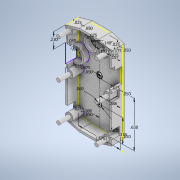
# Autodesk Inventor part: Back half gearbox
Saved by Autodesk Inventor 2020 (Build 240168000, 168)
## iProperties
Created: 2022-05-09
Part Number: Back half gearbox
Material: Generic
Document SubType Name: Modeling
Designer: Administrator
Density: 1 g/cm^3
Appearance: Default
Author: Administrator
Autodesk Inventor part; units mm, degrees
ref_plane "YZ Plane" through (0, 0, 0) normal (1, 0, 0) x (0, 1, 0)
ref_plane "XZ Plane" through (0, 0, 0) normal (0, 1, 0) x (-1, 0, 0)
ref_plane "XY Plane" through (0, 0, 0) normal (0, 0, 1) x (1, 0, 0)
sketch "Sketch1" plane through (0, 0, 0) normal (0, 0, 1) x (1, 0, 0)
  line L0 (-4.445, 2.3537) -> (-11.2171, 2.3537)
  line L1 (-16.0528, 3.6237) -> (-16.0528, 32.5162)
  line L2 (-11.2171, 33.8978) -> (-4.445, 33.8978)
  line L3 (0, 32.5162) -> (0, 3.6237)
  line L4 (-16.0528, 32.5162) -> (-11.2171, 33.8978)
  line L5 (-4.445, 33.8978) -> (0, 32.5162)
  line L6 (-16.0528, 3.6237) -> (-11.2171, 2.3537)
  line L7 (-4.445, 2.3537) -> (0, 3.6237)
  point P0 (0, 0)
  dimension "d13" = 28.8925
  dimension "d14" = 16.0528
  dimension "d15" = 28.8925
  dimension "d16" = 1.27
  dimension "d17" = 4.445
  constraints: 16 end point, 2 parallel, 2 vertical alignment, 1 horizontal, 1 horizontal alignment, 1 perpendicular
  measures "d13" distance of L3.start L3.end
  measures "d14" distance between parallel lines of L3 L1
  measures "d15" distance of L1.start L1.end
  measures "d16" distance from line of L0 L3.end
  measures "d17" distance from line of L3 L0.start
extrude "Extrusion1" add sketch "Sketch1" along normal blind 4.572
shell "Shell1" thickness 0.7112 removed faces 1 at (-8.9597, 23.3831, 4.572)
sketch "Sketch2" plane through (-11.1253, 3.0649, 0.7112) normal (0, 0, 1) x (1, 0, 0)
  circle A0 centre (3.0989, 7.3888) radius 0.762
  line L0 (-0.0918, -0.7112) -> (6.6803, -0.7112) projected
  line L1 (10.4141, 28.9276) -> (10.4141, 1.0953) projected
  line L2 (-4.2163, 1.1073) -> (-4.2163, 28.9148) projected
  circle A1 centre (3.0989, 16.2433) radius 0.9525
  line L3 (11.1253, 0.5588) -> (11.1253, 29.4513) projected
  line L4 (6.6803, -0.7112) -> (11.1253, 0.5588) projected
  line L5 (6.6803, 30.8329) -> (-0.0918, 30.8329) projected
  line L6 (-4.9275, 29.4513) -> (-4.9275, 0.5588) projected
  line L7 (3.0989, 30.8329) -> (3.0989, 0) construction
  line L8 (6.5806, 0) -> (0, 0) projected
  circle A2 centre (-3.2765, 20.0769) radius 0.762
  circle A3 centre (1.8543, 26.0069) radius 0.889
  circle A4 centre (6.4263, 25.6259) radius 0.762
  circle A5 centre (6.4263, 25.6259) radius 1.524
  arc A6 (0.4506, 27.0982) -> (1.8543, 27.7849) centre (1.8543, 26.0069) ccw
  arc A7 (-0.0507, 27.488) -> (1.8543, 28.4199) centre (1.8543, 26.0069) ccw
  line L9 (0.0078, 30.1217) -> (6.5723, 30.1217) projected
  line L10 (1.8543, 28.4199) -> (1.8543, 27.7849)
  line L11 (-0.0507, 27.488) -> (0.4506, 27.0982)
  line L12 (0.4506, 27.0982) -> (1.8456, 26.0137) construction
  arc A8 (-4.2163, 17.4457) -> (-4.2163, 22.7081) centre (-3.2765, 20.0769) ccw
  arc A9 (-4.2163, 18.1332) -> (-4.2163, 22.0206) centre (-3.2765, 20.0769) ccw
  point P0 (11.1253, -3.0649)
  point P1 (3.0989, 15.2908)
  point P2 (9.4743, 0.0871)
  dimension "d71" = 1.905
  dimension "d18" = 1.524
  dimension "d19" = 8.1
  dimension "d53" = 7.3152
  dimension "d54" = 14.6304
  dimension "d72" = 16.002
  dimension "d93" = 7.3152
  dimension "d98" = 3.556
  dimension "d99" = 0.635
  dimension "d100" = 4.572
  dimension "d101" = 0.381
  dimension "d102" = 3.9878
  dimension "d103" = 4.4958
  dimension "d104" = 1.905
  dimension "d105" = 2.032
  dimension "d106" = 0.635
  constraints: 9 centre point, 8 end point, 8 point on circle, 8 point on line, 4 vertical alignment, 1 coincident, 1 collinear, 1 vertical, 2 other
  measures "d18" diameter of A0
  measures "d19" distance from line of L0 A0.centre
  measures "d53" distance from line of L1 A0.centre
  measures "d54" distance between parallel lines of L1 L2
  measures "d72" distance from line of L0 point (3.099, 15.291)
  measures "d93" distance between parallel lines of L2 L7
  measures "d98" diameter of A6
  measures "d99" radial gap between concentric circles of A6 A7
  measures "d100" horizontal distance of A4.centre A6.centre
  measures "d101" vertical distance of A4.centre A3.centre
  measures "d102" distance from line of L1 A4.centre
  measures "d103" distance from line of L9 A4.centre
  measures "d104" horizontal distance of L10.start L11.start
  measures "d105" radial gap between concentric circles of A2 A8
  measures "d106" radial gap between concentric circles of A8 A9
sketch "Sketch3" plane through (-11.1253, 3.0649, 0.7112) normal (0, 0, 1) x (1, 0, 0)
  line L0 (6.5806, 0) -> (10.4141, 1.0953) projected
  line L1 (-4.2163, 1.1073) -> (0, 0) projected
  line L2 (10.4141, 28.9276) -> (10.4141, 1.0953) projected
  line L3 (-4.2163, 28.9148) -> (-4.2163, 1.1073) projected
  line L4 (6.5806, 0) -> (0, 0) construction
  circle A0 centre (9.7791, 15.2046) radius 0.635
  circle A1 centre (9.7791, 15.2046) radius 1.27
  circle A2 centre (-3.5813, 15.2046) radius 0.635
  circle A3 centre (-3.5813, 15.2046) radius 1.27
  line L5 (-4.2163, 1.1073) -> (-4.2163, 28.9148) projected
  circle A4 centre (-3.5813, 2.2053) radius 0.635
  circle A5 centre (-3.5813, 2.2053) radius 1.27
  circle A6 centre (9.7791, 2.2053) radius 0.635
  circle A7 centre (9.7791, 2.2053) radius 1.27
  circle A8 centre (-3.5813, 28.4359) radius 0.635
  circle A9 centre (-3.5813, 28.4359) radius 1.27
  circle A10 centre (9.7791, 28.46) radius 0.635
  circle A11 centre (9.7791, 28.46) radius 1.27
  line L6 (6.5723, 30.1217) -> (10.4141, 28.9276) projected
  line L7 (-4.2163, 28.9148) -> (0.0078, 30.1217) projected
  point P0 (11.1253, -3.0649)
  point P1 (10.4141, 16.3045)
  point P2 (10.4141, 14.1048)
  point P3 (10.4141, 15.2046)
  point P4 (-4.2163, 16.3045)
  point P5 (-4.2163, 15.2046)
  point P6 (-4.2163, 14.1048)
  point P7 (10.4141, 2.2053)
  point P8 (10.4141, 3.3052)
  point P9 (9.8642, 0.9382)
  point P10 (10.3762, 1.0844)
  point P11 (10.4141, 1.1055)
  point P12 (-3.5619, 0.9355)
  point P13 (-4.2163, 3.3052)
  point P14 (-4.2163, 2.2053)
  point P15 (9.9675, 29.0664)
  point P16 (8.9172, 29.3928)
  point P17 (10.4141, 27.3602)
  point P18 (10.4141, 28.46)
  point P19 (-2.6983, 29.3486)
  point P20 (-3.7558, 29.0464)
  point P21 (-4.2163, 28.4359)
  point P22 (-4.2163, 27.336)
  dimension "d57" = 1.27
  dimension "d58" = 0.635
  dimension "d59" = 1.27
  dimension "d60" = 0.635
  dimension "d63" = 1.27
  dimension "d64" = 0.635
  dimension "d65" = 1.27
  dimension "d66" = 0.635
  dimension "d67" = 1.27
  dimension "d68" = 0.635
  dimension "d69" = 1.27
  dimension "d70" = 0.635
  constraints: 12 centre point, 8 tangent
  measures "d57" diameter of A0
  measures "d58" radial gap between concentric circles of A0 A1
  measures "d59" diameter of A2
  measures "d60" radial gap between concentric circles of A2 A3
  measures "d63" diameter of A4
  measures "d64" radial gap between concentric circles of A4 A5
  measures "d65" diameter of A6
  measures "d66" radial gap between concentric circles of A6 A7
  measures "d67" diameter of A8
  measures "d68" radial gap between concentric circles of A8 A9
  measures "d69" diameter of A10
  measures "d70" radial gap between concentric circles of A10 A11
extrude "Extrusion10" add sketch "Sketch3" along normal blind 7.7216 contours A6 | A0 | A10 | A4 | A2 | A8
extrude "Extrusion11" cut sketch "Sketch2" against normal up to surface (0.7112 mm away) contours A0 | A1 | A2 | A3 | A4
extrude "Extrusion12" add sketch "Sketch2" along normal blind 1.905 contours L2 A9 A8 | A5 | A6 L10 A7 L11
sketch "Sketch5" plane through (-16.0528, 3.6237, 0) normal (-1, 0, 0) x (0, 0, 1)
  line L0 (4.572, 14.6458) -> (4.572, 27.8771) projected
  line L1 (4.572, 23.5585) -> (3.302, 23.5585)
  line L2 (3.302, 13.3985) -> (4.572, 13.3985)
  line L3 (0, 28.8925) -> (4.572, 28.8925) projected
  line L4 (3.302, 22.4155) -> (0.7112, 22.4155)
  line L5 (1.778, 13.3985) -> (3.302, 13.3985)
  line L6 (1.778, 15.9385) -> (1.778, 13.3985)
  line L7 (4.572, 15.9385) -> (1.778, 15.9385)
  line L8 (0.7112, 17.0815) -> (4.572, 17.0815)
  line L9 (3.302, 23.5585) -> (3.302, 22.4155)
  line L10 (4.572, 13.3985) -> (4.572, 15.9385)
  line L11 (4.572, 17.0815) -> (4.572, 23.5585)
  line L12 (0.7112, 22.3121) -> (0.7112, 16.7241) projected
  line L13 (0.7112, 17.0815) -> (0.7112, 22.4155)
  point P0 (0, -3.6237)
  point P1 (0.7112, 22.1493)
  point P2 (0.7112, 16.8869)
  dimension "d109" = 5.334
  dimension "d114" = 1.143
  constraints: 22 end point, 5 parallel, 3 horizontal, 2 perpendicular, 2 point on line, 1 collinear
  measures "d109" distance between parallel lines of L3 L1
  measures "d114" distance between parallel lines of L4 L1
extrude "Extrusion14" add sketch "Sketch3" along normal up to surface (3.8608 mm away) contours A6 | A7 L2 L0 | A11 L6 A10 L2 | L2 L6 A11 | A0 | A1 L2 | L0 A7 | A7 L2 | A10 L6 L2 | A10 | A4 | L3 A5 L1 | A5 L3 | A9 L7 L3 | L3 A8 L7 A9 | A3 L3 | A2 | L3 A3 | L1 A5 | L3 L7 A8 | A8 picked at (10.0816, 1.2114) picked at (10.1817, 14.2329)
extrude "Extrusion13" cut sketch "Sketch5" against normal up to surface (0.7112 mm away)
extrude "Extrusion15" cut sketch "Sketch5" along normal up to surface (0.7112 mm away) from surface at -16.0528
sketch "Sketch6" plane through (0, 0, 4.572) normal (0, 0, 1) x (1, 0, 0)
  line L0 (-0.7112, 6.37) -> (-0.7112, 17.1697) projected
  line L1 (0, 8.275) -> (-0.7112, 8.275)
  line L2 (-0.7112, 8.275) -> (-0.7112, 6.37)
  line L3 (0, 6.37) -> (0, 8.275)
  arc A0 (-0.7112, 6.37) -> (-1.261, 4.003) centre (-1.3462, 5.2702) ccw projected
  circle A1 centre (-14.7066, 5.2702) radius 0.635 projected
  arc A2 (-0.7491, 4.1493) -> (-0.7112, 4.1703) centre (-1.3462, 5.2702) ccw projected
  line L4 (-0.7112, 4.1703) -> (-0.7112, 4.1601) projected
  line L5 (-0.7112, 4.1601) -> (-0.7491, 4.1493) projected
  circle A3 centre (-1.3462, 5.2702) radius 0.635 projected
  line L6 (0, 17.0222) -> (-0.7112, 17.0222) projected
  line L7 (-0.7112, 17.0222) -> (-0.7112, 6.37) projected
  arc A4 (-0.7112, 6.37) -> (-1.261, 4.003) centre (-1.3462, 5.2702) ccw projected
  line L8 (-1.261, 4.003) -> (-4.5446, 3.0649) projected
  line L9 (-4.5446, 3.0649) -> (-11.1253, 3.0649) projected
  line L10 (-11.1253, 3.0649) -> (-14.6871, 4.0003) projected
  arc A5 (-14.6871, 4.0003) -> (-15.3416, 6.37) centre (-14.7066, 5.2702) ccw projected
  line L11 (-15.3416, 6.37) -> (-15.3416, 17.0222) projected
  line L12 (-15.3416, 17.0222) -> (-16.0528, 17.0222) projected
  line L13 (-16.0528, 17.0222) -> (-16.0528, 3.6237) projected
  line L14 (-16.0528, 3.6237) -> (-11.2171, 2.3537) projected
  line L15 (-11.2171, 2.3537) -> (-4.445, 2.3537) projected
  line L16 (-4.445, 2.3537) -> (0, 3.6237) projected
  line L17 (0, 3.6237) -> (0, 17.0222) projected
  arc A6 (-0.7112, 6.37) -> (-1.261, 4.003) centre (-1.3462, 5.2702) ccw construction
  circle A7 centre (-1.3462, 5.2702) radius 1.27 construction
  arc A8 (0, 5.4827) -> (-0.7112, 6.37) centre (-1.4943, 5.0137) ccw
  line L18 (0, 6.37) -> (0, 5.4827)
  line L19 (-8.0264, 33.8978) -> (-8.0264, 3.0649) construction
  line L20 (-16.0528, 8.275) -> (-15.3416, 8.275)
  line L21 (-16.0528, 6.37) -> (-16.0528, 8.275)
  line L22 (-15.3416, 8.275) -> (-15.3416, 6.37)
  line L23 (-16.0528, 5.4827) -> (-16.0528, 8.275)
  arc A9 (-15.3416, 6.37) -> (-16.0528, 5.4827) centre (-14.5585, 5.0137) ccw
  line L24 (-16.0528, 6.37) -> (-16.0528, 5.4827)
  point P0 (0, 0)
  constraints: 18 end point, 6 symmetric about line, 4 point on circle, 3 centre point, 1 coincident, 1 collinear, 1 horizontal, 1 parallel, 1 perpendicular, 1 point on line, 1 tangent, 1 other
extrude "Extrusion16" cut sketch "Sketch6" against normal up to surface (2.794 mm away) contours L0 L1 L3 L17 A8 | A9 L13 L20 L11
body "Solid1"
